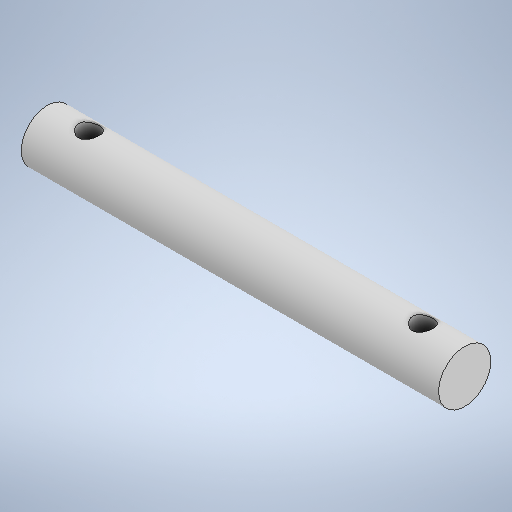
# Autodesk Inventor part: TIE ROD
Saved by Autodesk Inventor 2025 (Build 290162010, 162A)
## iProperties
Created: 2024-08-09
Part Number: TIE ROD
Material: Generic
Document SubType Name: Modeling
Designer: darkb
Density: 1 g/cm^3
Appearance: Default
Author: darkb
Autodesk Inventor part; units mm, degrees
ref_plane "YZ Plane" through (0, 0, 0) normal (1, 0, 0) x (0, 1, 0)
ref_plane "XZ Plane" through (0, 0, 0) normal (0, 1, 0) x (-1, 0, 0)
ref_plane "XY Plane" through (0, 0, 0) normal (0, 0, 1) x (1, 0, 0)
sketch "Sketch1" plane through (0, 0, 0) normal (1, 0, 0) x (0, 1, 0)
  circle A0 centre (0, 0) radius 3.175
  dimension "d0" = 6.35
  constraints: 1 centre point, 1 coincident
  measures "d0" diameter of A0
extrude "Extrusion1" add sketch "Sketch1" along normal blind 50.8
sketch "Sketch2" plane through (0, 0, 0) normal (0, 1, 0) x (-1, 0, 0)
  circle A0 centre (-5.08, 0) radius 1.27
  line L0 (0, 3.175) -> (0, -3.175) projected
  point P0 (0, 0)
  dimension "d3" = 2.54
  dimension "d4" = 5.08
  constraints: 1 centre point
  measures "d3" diameter of A0
  measures "d4" distance from line of L0 A0.centre
extrude "Extrusion2" cut sketch "Sketch2" along normal mid plane 50.8
sketch "Sketch3" plane through (0, 0, 0) normal (0, 1, 0) x (-1, 0, 0)
  circle A0 centre (-45.72, 0) radius 1.27
  line L0 (-50.8, 3.175) -> (-50.8, -3.175) projected
  point P0 (0, 0)
  dimension "d7" = 2.54
  dimension "d8" = 5.08
  constraints: 1 centre point
  measures "d7" diameter of A0
  measures "d8" distance from line of L0 A0.centre
extrude "Extrusion3" cut sketch "Sketch3" along normal mid plane 50.8
body "Solid1"
